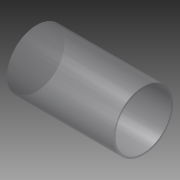
# Autodesk Inventor part: MainTube
Saved by Autodesk Inventor 2015 (Build 190159000, 159)
## iProperties
Created: 2014-07-23
Part Number: MainTube
Material: PET Plastic
Document SubType Name: Modeling
Designer: STACKPOLE
Density: 1.541 g/cm^3
Mass: 253.582 g
Surface Area: 1115.33 cm^2
Volume: 164.557 cm^3
Appearance: Polycarbonate - Clear
Author: STACKPOLE
Autodesk Inventor part; units mm, degrees
ref_plane "YZ Plane" through (0, 0, 0) normal (1, 0, 0) x (0, 1, 0)
ref_plane "XZ Plane" through (0, 0, 0) normal (0, 1, 0) x (-1, 0, 0)
ref_plane "XY Plane" through (0, 0, 0) normal (0, 0, 1) x (1, 0, 0)
sketch "Sketch1" plane through (0, 0, 0) normal (1, 0, 0) x (0, 1, 0)
  circle A0 centre (0, 0) radius 50
  circle A1 centre (0, 0) radius 47
  dimension "d0" = 100
  dimension "d2" = 94
  constraints: 2 centre point, 2 coincident
  measures "d0" diameter of A0
  measures "d2" diameter of A1
extrude "Extrusion1" add sketch "Sketch1" along normal blind 180
body "Solid1"
